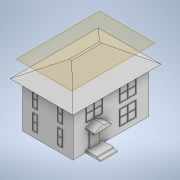
# Autodesk Inventor part: villa1
Saved by Autodesk Inventor 2020 (Build 240168000, 168)
## iProperties
Created: 2021-10-28
Part Number: villa1
Material: 常规
Document SubType Name: Modeling
Designer: mhn
Density: 1 g/cm^3
Appearance: 默认
Author: mhn
Autodesk Inventor part; units mm, degrees
ref_plane "YZ Plane" through (0, 0, 0) normal (1, 0, 0) x (0, 1, 0)
ref_plane "XZ Plane" through (0, 0, 0) normal (0, 1, 0) x (-1, 0, 0)
ref_plane "XY Plane" through (0, 0, 0) normal (0, 0, 1) x (1, 0, 0)
sketch "草图1" plane through (0, 0, 0) normal (0, 1, 0) x (-1, 0, 0)
  line L0 (-100, 150) -> (100, 150)
  line L1 (100, 150) -> (100, -150)
  line L2 (100, -150) -> (-100, -150)
  line L3 (-100, -150) -> (-100, 150)
  line L4 (-100, 150) -> (100, -150) construction
  line L5 (100, 150) -> (-100, -150) construction
  point P0 (0, 0)
  dimension "d0" = 300
  dimension "d1" = 200
  constraints: 12 end point, 2 midpoint, 2 parallel, 1 horizontal, 1 perpendicular
  measures "d0" distance of L0.end L1.end
  measures "d1" distance of L1.end L2.end
extrude "拉伸1" add sketch "草图1" along normal blind 180
sketch "草图2" plane through (0, 180, 0) normal (0, 1, 0) x (1, 0, 0)
  line L0 (125, -175) -> (-125, -175)
  line L1 (-125, -175) -> (-125, 175)
  line L2 (-125, 175) -> (125, 175)
  line L3 (125, 175) -> (125, -175)
  line L4 (125, -175) -> (-125, 175) construction
  line L5 (-125, -175) -> (125, 175) construction
  point P0 (0, 0)
  dimension "d4" = 350
  dimension "d5" = 250
  constraints: 12 end point, 2 midpoint, 2 parallel, 1 horizontal, 1 perpendicular
  measures "d4" distance of L0.end L1.end
  measures "d5" distance of L1.end L2.end
ref_plane "工作平面1" through (0, 250, 0) normal (0, 1, 0) x (1, 0, 0)
sketch "草图3" plane through (0, 250, 0) normal (0, 1, 0) x (1, 0, 0)
  line L0 (-5, -60) -> (5, -60)
  line L1 (5, -60) -> (5, 60)
  line L2 (5, 60) -> (-5, 60)
  line L3 (-5, 60) -> (-5, -60)
  line L4 (-5, -60) -> (5, 60) construction
  line L5 (5, -60) -> (-5, 60) construction
  point P0 (0, 0)
  dimension "d9" = 120
  dimension "d10" = 10
  constraints: 12 end point, 2 midpoint, 2 parallel, 1 horizontal, 1 perpendicular
  measures "d9" distance of L2.end L0.start
  measures "d10" distance of L1.end L2.end
loft "放样1" add profiles "草图2", "草图3"
sketch "草图4" plane through (100, 0, -150) normal (0, 0, -1) x (-1, 0, 0)
  line L0 (40, 164.7987) -> (60, 164.7987)
  line L1 (60, 164.7987) -> (60, 102.7987)
  line L2 (60, 102.7987) -> (40, 102.7987)
  line L3 (40, 102.7987) -> (40, 164.7987)
  line L4 (42, 162.7987) -> (58, 162.7987)
  line L5 (58, 162.7987) -> (58, 135.7987)
  line L6 (58, 135.7987) -> (42, 135.7987)
  line L7 (42, 135.7987) -> (42, 162.7987)
  line L8 (42, 133.7987) -> (58, 133.7987)
  line L9 (58, 133.7987) -> (58, 104.7987)
  line L10 (58, 104.7987) -> (42, 104.7987)
  line L11 (42, 104.7987) -> (42, 133.7987)
  line L12 (0, 0) -> (0, 180) projected
  point P0 (100, 0)
  dimension "d15" = 62
  dimension "d16" = 2
  dimension "d17" = 2
  dimension "d18" = 2
  dimension "d19" = 2
  dimension "d20" = 2
  dimension "d21" = 20
  dimension "d22" = 29
  dimension "d23" = 40
  constraints: 24 end point, 6 parallel, 3 horizontal, 3 perpendicular, 2 point on line
  measures "d15" distance of L0.end L1.end
  measures "d16" distance between parallel lines of L1 L5
  measures "d17" distance between parallel lines of L3 L7
  measures "d18" distance between parallel lines of L4 L0
  measures "d19" distance between parallel lines of L8 L6
  measures "d20" distance between parallel lines of L2 L10
  measures "d21" distance of L0.start L0.end
  measures "d22" distance of L8.end L9.end
  measures "d23" distance between parallel lines of L12 L3
extrude "拉伸2" add sketch "草图4" along normal blind 2
pattern_linear "矩形阵列1" count 2 spacing 80 along (0, -1, 0) count 2 spacing 100 along (-1, 0, 0) of "拉伸2"
mirror "镜像1" about plane through (0, 0, 0) normal (0, 0, 1) of "拉伸2", "矩形阵列1"
sketch "草图5" plane through (100, 0, 150) normal (1, 0, 0) x (0, 0, -1)
  line L0 (50, 84.7987) -> (116, 84.7987)
  line L1 (116, 84.7987) -> (83, 99.7987)
  line L2 (50, 84.7987) -> (83, 99.7987)
  line L3 (50, 84.7987) -> (116, 84.7987)
  line L4 (116, 84.7987) -> (116, 80.7987)
  line L5 (116, 80.7987) -> (50, 80.7987)
  line L6 (50, 80.7987) -> (50, 84.7987)
  line L7 (0, 0) -> (0, 180) projected
  point P0 (150, 0)
  dimension "d32" = 66
  dimension "d33" = 15
  dimension "d34" = 33
  dimension "d35" = 4
  dimension "d60" = 50
  dimension "d61" = 66
  constraints: 15 end point, 2 horizontal, 2 parallel, 1 perpendicular
  measures "d32" distance of L0.start L0.end
  measures "d33" distance from line of L1.end L0
  measures "d34" horizontal distance of L1.end L0.end
  measures "d35" distance of L3.end L4.end
  measures "d60" distance from line of L7 L0.start
  measures "d61" distance of L4.end L5.end
extrude "拉伸3" add sketch "草图5" along normal blind 35
sketch "草图6" plane through (100, 80.7987, 34) normal (0, 0, -1) x (-1, 0, 0)
  line L0 (0, -80.7987) -> (0, 99.2013) projected
  line L1 (0, -80.7987) -> (-60, -80.7987)
  line L2 (-60, -80.7987) -> (-60, -75.7987)
  line L3 (-60, -75.7987) -> (0, -75.7987)
  line L4 (0, -75.7987) -> (0, -80.7987)
  line L5 (0, -75.7987) -> (-45, -75.7987)
  line L6 (-45, -75.7987) -> (-45, -70.7987)
  line L7 (-45, -70.7987) -> (0, -70.7987)
  line L8 (0, -70.7987) -> (0, -75.7987)
  point P0 (100, -80.7987)
  point P1 (0, -70.7987)
  dimension "d38" = 5
  dimension "d39" = 5
  dimension "d40" = 45
  dimension "d41" = 60
  constraints: 16 end point, 4 parallel, 2 horizontal, 2 perpendicular
  measures "d38" distance of L1.end L2.end
  measures "d39" distance of L5.end L6.end
  measures "d40" distance of L6.end L7.end
  measures "d41" distance of L0.start L1.end
extrude "拉伸4" add sketch "草图6" against normal blind 66
sketch "草图7" plane through (100, 0, -150) normal (1, 0, 0) x (0, 0, -1)
  line L0 (-50, 103.2655) -> (-116, 103.2655)
  line L1 (-116, 103.2655) -> (-116, 163.2655)
  line L2 (-116, 163.2655) -> (-50, 163.2655)
  line L3 (-50, 163.2655) -> (-50, 103.2655)
  line L4 (-114, 161.2655) -> (-84, 161.2655)
  line L5 (-84, 161.2655) -> (-84, 134.2655)
  line L6 (-84, 134.2655) -> (-114, 134.2655)
  line L7 (-114, 134.2655) -> (-114, 161.2655)
  line L8 (-82, 161.2655) -> (-52, 161.2655)
  line L9 (-52, 161.2655) -> (-52, 134.2655)
  line L10 (-52, 134.2655) -> (-82, 134.2655)
  line L11 (-82, 134.2655) -> (-82, 161.2655)
  line L12 (-52, 132.2655) -> (-82, 132.2655)
  line L13 (-82, 132.2655) -> (-82, 105.2655)
  line L14 (-82, 105.2655) -> (-52, 105.2655)
  line L15 (-52, 105.2655) -> (-52, 132.2655)
  line L16 (-84, 105.2655) -> (-114, 105.2655)
  line L17 (-114, 105.2655) -> (-114, 132.2655)
  line L18 (-114, 132.2655) -> (-84, 132.2655)
  line L19 (-84, 132.2655) -> (-84, 105.2655)
  line L20 (0, 0) -> (0, 180) projected
  point P0 (-150, 0)
  dimension "d44" = 66
  dimension "d45" = 60
  dimension "d46" = 2
  dimension "d47" = 2
  dimension "d48" = 2
  dimension "d49" = 2
  dimension "d50" = 2
  dimension "d51" = 2
  dimension "d52" = 30
  dimension "d53" = 27
  dimension "d54" = 50
  constraints: 40 end point, 10 parallel, 8 point on line, 5 horizontal, 5 perpendicular
  measures "d44" distance of L1.end L2.end
  measures "d45" distance of L0.end L1.end
  measures "d46" distance between parallel lines of L4 L2
  measures "d47" distance between parallel lines of L1 L7
  measures "d48" distance between parallel lines of L6 L18
  measures "d49" distance between parallel lines of L0 L16
  measures "d50" distance between parallel lines of L3 L9
  measures "d51" distance between parallel lines of L5 L11
  measures "d52" distance of L8.start L8.end
  measures "d53" distance of L10.end L8.start
  measures "d54" distance between parallel lines of L3 L20
extrude "拉伸5" add sketch "草图7" along normal blind 2
pattern_linear "矩形阵列2" count 2 spacing 80 along (0, -1, 0) of "拉伸5"
mirror "镜像2" about plane through (0, 0, 0) normal (1, 0, 0) of "拉伸5", "矩形阵列2"
mirror "镜像3" about plane through (0, 0, 0) normal (0, 0, 1) of "拉伸5", "矩形阵列2", "镜像2"
sketch "草图8" plane through (100, 0, -150) normal (1, 0, 0) x (0, 0, -1)
  line L0 (-250, 23.2655) -> (-250, 83.2655) projected
  line L1 (-184, 23.2655) -> (-184, 83.2655) projected
  line L2 (-184, 80.4641) -> (-184, 23.2655)
  line L3 (-184, 23.2655) -> (-250, 23.2655)
  line L4 (-250, 23.2655) -> (-250, 80.4641)
  line L5 (-250, 80.7987) -> (-184, 80.7987) projected
  point P0 (-150, 0)
  constraints: 6 end point, 1 parallel, 1 point on line
extrude "拉伸6" cut sketch "草图8" along normal blind 4
sketch "草图9" plane through (100, 0, -150) normal (1, 0, 0) x (0, 0, -1)
  line L0 (-184, 10) -> (-250, 10) projected
  line L1 (-237, 10) -> (-197, 10)
  line L2 (-197, 10) -> (-197, 70)
  line L3 (-197, 70) -> (-237, 70)
  line L4 (-237, 70) -> (-237, 10)
  line L5 (-227, 62) -> (-207, 62)
  line L6 (-207, 62) -> (-207, 52)
  line L7 (-207, 52) -> (-227, 52)
  line L8 (-227, 52) -> (-227, 62)
  line L9 (-184, 10) -> (-184, 5) projected
  point P0 (-150, 0)
  dimension "d64" = 40
  dimension "d65" = 60
  dimension "d66" = 10
  dimension "d67" = 20
  dimension "d68" = 10
  dimension "d69" = 8
  dimension "d70" = 13
  constraints: 16 end point, 4 parallel, 2 horizontal, 2 perpendicular, 1 point on line
  measures "d64" distance of L2.end L3.end
  measures "d65" distance of L1.end L2.end
  measures "d66" distance of L5.end L6.end
  measures "d67" distance of L5.start L5.end
  measures "d68" distance between parallel lines of L2 L6
  measures "d69" distance between parallel lines of L3 L5
  measures "d70" distance from line of L9 L1.end
extrude "拉伸7" add sketch "草图9" along normal blind 4
